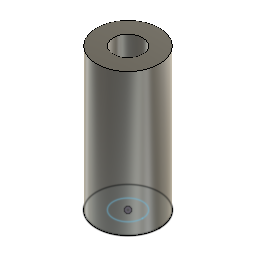
syringe-adapter v3 (Autodesk Fusion 360 design; units mm, degrees)
Autodesk Fusion 360 part; units mm, degrees
sketch "Sketch2" plane through (0, 0, 0) normal (0, 0, 1) x (1, 0, 0)
  circle A0 centre (0, 0) radius 2.25
  dimension "d2" = 4.5
  constraint coincident A0.centre origin
  measures "d2" diameter of A0
ref_plane "WorkPlane1" through (0, 0, 8.1) normal (0, 0, 1) x (1, 0, 0)
sketch "Sketch3" plane through (0, 0, 8.1) normal (0, 0, 1) x (1, 0, 0)
  circle A0 centre (0, 0) radius 2.05
  dimension "d5" = 4.1
  constraint coincident A0.centre origin
  measures "d5" diameter of A0
loft "Loft1" add profiles "Sketch3", "Sketch2" section 1 section 2 makes body 1
sketch "Sketch4" plane through (0, 0, 0) normal (0, 0, 1) x (1, 0, 0)
  circle A0 centre (0, 0) radius 4.4
  circle A1 centre (0, 0) radius 2.05
  dimension "d6" = 8.8
  dimension "d9" = 4.1
  constraint coincident A0.centre A1.centre
  measures "d6" diameter of A0
  measures "d9" diameter of A1
extrude "Extrude1" add sketch "Sketch4" along normal blind 20 separate body contours A0 | A1 makes body 2
combine "Combine1" operation cut target body 2 tool bodies 1 keep tools
extrude "Extrude2" cut sketch "Sketch4" along normal blind 40 contours A1 bodies 2
hidden bodies 1
named bodies: "neg tip", "outer"
